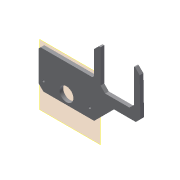
# Autodesk Inventor part: 10_MiniSPIM_XY_Stageplate
Saved by Autodesk Inventor 2019 (Build 230136000, 136)
## iProperties
Created: 2019-10-17
Part Number: 10_MiniSPIM_XY_Stageplate
Material: Generic
Document SubType Name: Modeling
Designer: diederichbenedict
Density: 1 g/cm^3
Appearance: Default
Author: diederichbenedict
Autodesk Inventor part; units mm, degrees
ref_plane "YZ Plane" through (0, 0, 0) normal (1, 0, 0) x (0, 1, 0)
ref_plane "XZ Plane" through (0, 0, 0) normal (0, 1, 0) x (-1, 0, 0)
ref_plane "XY Plane" through (0, 0, 0) normal (0, 0, 1) x (1, 0, 0)
ref_plane "Work Plane1" through (0, 0, 0) normal (0, 0, 1) x (1, 0, 0)
sketch "Sketch1" plane through (0, 0, 0) normal (0, 0, 1) x (1, 0, 0)
  line L0 (28, 30) -> (30, 28) projected
  line L1 (28, 30) -> (-28, 30) projected
  line L2 (-30, 28) -> (-28, 30) projected
  line L3 (-30, 28) -> (-30, -28) projected
  line L4 (-28, -30) -> (-30, -28) projected
  line L5 (-28, -30) -> (28, -30) projected
  line L6 (30, -28) -> (28, -30) projected
  line L7 (30, -28) -> (30, 28) projected
  circle A0 centre (25, 0) radius 1.3 projected
  circle A1 centre (-25, 0) radius 1.3 projected
  circle A2 centre (0, 0) radius 7.5 projected
  line L8 (-30, -9.9552) -> (30, -9.9552)
  line L9 (30, -9.9552) -> (51.4888, 11.5337)
  line L10 (30, -9.9552) -> (60.3898, -9.9552) construction
  line L11 (51.4888, 11.5337) -> (80.0964, 11.5337)
  line L12 (80.0964, 11.5337) -> (79.2136, 62.4273)
  line L13 (79.2136, 62.4273) -> (30, 62.4273)
  line L14 (30, 62.4273) -> (30, 32)
  line L15 (30, 32) -> (28, 30)
  line L16 (30, 7.5) -> (36.7448, 7.5)
  line L17 (36.7448, 7.5) -> (36.7448, 17.9412)
  line L18 (36.7448, 17.9412) -> (73.91, 17.9412)
  line L19 (73.91, 17.9412) -> (73.91, 58.2218)
  line L20 (73.91, 58.2218) -> (36.7448, 58.2218)
  line L21 (36.7448, 58.2218) -> (36.7448, 32)
  line L22 (36.7448, 32) -> (36.7448, 17.9412)
  circle A3 centre (43.1, 13.7082) radius 0.9 projected
  circle A4 centre (70.1, 14.5773) radius 0.9 projected
  circle A5 centre (59.8, 60.4273) radius 0.9 projected
  line L23 (52.7, 62.4273) -> (61.8, 62.4273) projected
  point P0 (0, 0)
  dimension "d0" = 45
  constraints: 30 end point, 6 perpendicular, 6 point on line, 3 horizontal, 2 parallel, 1 equal length, 1 vertical
  measures "d0" angle of L10 L9
extrude "Extrusion1" add sketch "Sketch1" along normal blind 4 contours L15 L14 L13 L12 L11 L9 L7 L0 | L0 L7 L8 L3 L2 L1 | L22 L21 L20 L19 L18 | A3 | A4 | A5
sketch "Sketch2" plane through (0, 0, 4) normal (0, 0, 1) x (1, 0, 0)
  circle A0 centre (43.1, 18.7082) radius 2.25
  circle A1 centre (59.8, 65.4273) radius 0.9 projected
  circle A2 centre (59.8, 65.4273) radius 3
  line L0 (79.2136, 62.4273) -> (30, 62.4273) projected
  circle A3 centre (70.1, 19.5773) radius 2
  circle A4 centre (43.1, 13.7082) radius 0.9
  circle A5 centre (70.1, 14.5773) radius 0.9
  circle A6 centre (59.8, 60.4273) radius 0.9
  point P0 (0, 0)
  dimension "d4" = 4.5
  dimension "d5" = 4
  constraints: 6 centre point, 1 coincident, 1 tangent, 6 other
  measures "d4" diameter of A0
  measures "d5" diameter of A3
ref_plane "Work Plane2" through (65, 14.0254, 8.3) normal (0, 0, 1) x (1, 0, 0)
ref_plane "Work Plane3" through (41, 13.4694, 7.3) normal (0, 0, -1) x (0, 1, 0)
extrude "Extrusion2" [suppressed]
sketch "Sketch3" plane through (59.8, 65.4273, 7.3) normal (0, 0, 1) x (1, 0, 0)
  circle A0 centre (0, 0) radius 3 projected
  circle A1 centre (0, 0) radius 0.9 projected
  point P0 (-59.8, -65.4273)
ref_plane "Work Plane4" through (52.7, 52.6273, 8.5) normal (0, 0, -1) x (0, 1, 0)
extrude "Extrusion3" [suppressed]
sketch "Sketch4" plane through (0, 0, 4) normal (0, 0, 1) x (1, 0, 0)
  arc A0 (45.1, 18.7082) -> (41.5, 19.9082) centre (43.1, 18.7082) ccw projected
  circle A1 centre (70.1, 19.5773) radius 2 projected
  circle A2 centre (59.8, 65.4273) radius 3 projected
  line L0 (73.1637, 21.5773) -> (36.8888, 21.5773)
  line L1 (36.8888, 21.5773) -> (36.8888, 63.4273)
  line L2 (36.8888, 63.4273) -> (73.1637, 63.4273)
  line L3 (73.1637, 63.4273) -> (73.1637, 21.5773)
  point P0 (0, 0)
  constraints: 8 end point, 2 parallel, 1 horizontal, 1 perpendicular
extrude "Extrusion4" cut sketch "Sketch4" against normal blind 4 contours L0 L1 L2 A2 L3 | A2 L2 picked at (59.2347, 63.2691)
chamfer "Chamfer1" distance 5 angle 45 6 edges at (36.8888, 21.5773, 2) (30, 62.4273, 2) (73.1637, 21.5773, 2) (79.2136, 62.4273, 2) (80.0964, 11.5337, 2) (-30, -9.9552, 2)
body "Solid1"
